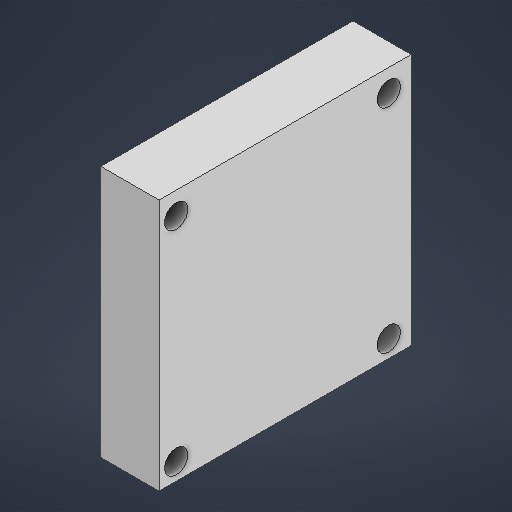
# Autodesk Inventor part: SAFRS-P-0005
Saved by Autodesk Inventor 2026.2 (Build 302298000, 298)
## iProperties
Created: 2025-11-26
Part Number: SAFRS-P-0005
Material: 일반
Document SubType Name: Modeling
Designer: jaewook
Density: 1 g/cm^3
Appearance: 기본값
Author: jaewook
Title: L298N Base
Autodesk Inventor part; units mm, degrees
ref_plane "YZ Plane" through (0, 0, 0) normal (1, 0, 0) x (0, 1, 0)
ref_plane "XZ Plane" through (0, 0, 0) normal (0, 1, 0) x (-1, 0, 0)
ref_plane "XY Plane" through (0, 0, 0) normal (0, 0, 1) x (1, 0, 0)
sketch "스케치1" plane through (0, 0, 0) normal (1, 0, 0) x (0, 1, 0)
  line L0 (-21.65, 21.65) -> (21.65, 21.65)
  line L1 (21.65, 21.65) -> (21.65, -21.65)
  line L2 (21.65, -21.65) -> (-21.65, -21.65)
  line L3 (-21.65, -21.65) -> (-21.65, 21.65)
  line L4 (-21.65, 21.65) -> (21.65, -21.65) construction
  line L5 (21.65, 21.65) -> (-21.65, -21.65) construction
  circle A0 centre (17.8, -17.8) radius 2
  line L6 (0, 0) -> (21.65, 0) construction
  line L7 (0, -21.65) -> (0, 0) construction
  circle A1 centre (17.8, 18.7) radius 2
  circle A2 centre (-18.7, -17.8) radius 2
  circle A3 centre (-18.7, 18.7) radius 2
  dimension "d0" = 43.3
  dimension "d1" = 43.3
  dimension "d4" = 4
  dimension "d5" = 17.8
  dimension "d8" = 36.5
  dimension "d11" = 36.5
  constraints: 16 end point, 4 centre point, 4 midpoint, 2 horizontal, 2 parallel, 2 vertical, 1 perpendicular, 1 point on line, 6 other
  measures "d0" distance of L1.end L2.end
  measures "d1" distance of L0.end L1.end
  measures "d4" diameter of A0
  measures "d5" distance from line of L6 A0.centre
  measures "d8" distance of A0.centre A1.centre
  measures "d11" distance of A0.centre A2.centre
extrude "돌출1" add sketch "스케치1" along normal blind 10
